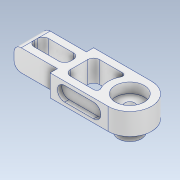
# Autodesk Inventor part: ServoArm
Saved by Autodesk Inventor 2020 (Build 240168000, 168)
## iProperties
Created: 2019-12-15
Part Number: ServoArm
Material: Aluminum 6061
Document SubType Name: Modeling
Designer: Kjell
Density: 2.7 g/cm^3
Appearance: Aluminum - Flat
Author: Kjell
Autodesk Inventor part; units mm, degrees
ref_plane "YZ Plane" through (0, 0, 0) normal (1, 0, 0) x (0, 1, 0)
ref_plane "XZ Plane" through (0, 0, 0) normal (0, 1, 0) x (-1, 0, 0)
ref_plane "XY Plane" through (0, 0, 0) normal (0, 0, 1) x (1, 0, 0)
ref_plane "Work Plane1" through (0, 0, 0) normal (0, 0, 1) x (1, 0, 0)
sketch "Sketch1" plane through (0, 0, 0) normal (0, 0, 1) x (1, 0, 0)
  arc A0 (-2.5, 4.5) -> (-4.5, 2.5) centre (-2.5, 2.5) ccw projected
  arc A1 (-2.5, 4.5) -> (-4.5, 2.5) centre (-2.5, 2.5) ccw projected
  line L0 (-2.5, 4.5) -> (2.5, 4.5) projected
  arc A2 (4.5, 2.5) -> (2.5, 4.5) centre (2.5, 2.5) ccw projected
  line L1 (4.5, 2.5) -> (4.5, -2.5) projected
  arc A3 (2.5, -4.5) -> (4.5, -2.5) centre (2.5, -2.5) ccw projected
  line L2 (2.5, -4.5) -> (-2.5, -4.5) projected
  arc A4 (-4.5, -2.5) -> (-2.5, -4.5) centre (-2.5, -2.5) ccw projected
  line L3 (-4.5, -2.5) -> (-4.5, 2.5) projected
  circle A5 centre (0, 0) radius 5.675 projected
  circle A6 centre (0, 0) radius 8
  circle A7 centre (0, 0) radius 6
  line L4 (-4.55, 2.5) -> (-4.55, -2.5)
  arc A8 (-4.55, -2.5) -> (-2.5, -4.55) centre (-2.5, -2.5) ccw
  line L5 (-2.5, -4.55) -> (2.5, -4.55)
  arc A9 (2.5, -4.55) -> (4.55, -2.5) centre (2.5, -2.5) ccw
  line L6 (4.55, -2.5) -> (4.55, 2.5)
  arc A10 (4.55, 2.5) -> (2.5, 4.55) centre (2.5, 2.5) ccw
  line L7 (2.5, 4.55) -> (-2.5, 4.55)
  point P0 (0, 0)
  dimension "d0" = 16
  dimension "d1" = 12
  dimension "d2" = 0.05
  constraints: 8 end point, 6 point on circle, 5 centre point, 2 coincident, 6 other
  measures "d0" diameter of A6
  measures "d1" diameter of A7
  measures "d2" distance between parallel lines of L2 L5
extrude "Extrusion1" add sketch "Sketch1" against normal blind 5 contours A5 | A6 | A7
sketch "Sketch2" plane through (0, 0, -5) normal (0, 0, -1) x (-1, 0, 0)
  circle A0 centre (0, 0) radius 8 projected
  circle A1 centre (0, 0) radius 6
  dimension "d5" = 12
  constraints: 1 centre point, 1 coincident
  measures "d5" diameter of A1
extrude "Extrusion2" add sketch "Sketch2" along normal blind 3
sketch "Sketch4" plane through (0, 0, 0) normal (0, 0, 1) x (1, 0, 0)
  circle A0 centre (0, 0) radius 8 projected
  arc A1 (0, -15) -> (0, 15) centre (0, 0) ccw
  line L0 (-70, -15) -> (0, -15)
  line L1 (0, 15) -> (-70, 15)
  line L2 (-70, 15) -> (-70, -15)
  line L3 (-30, -67.5) -> (30, -67.5) construction
  line L4 (30, -67.5) -> (30, 67.5) construction
  line L5 (30, 67.5) -> (-30, 67.5) construction
  line L6 (-30, 67.5) -> (-30, -67.5) construction
  line L7 (-30, -67.5) -> (30, 67.5) construction
  line L8 (30, -67.5) -> (-30, 67.5) construction
  dimension "d10" = 30
  dimension "d11" = 60
  dimension "d12" = 135
  dimension "ArmLength" = 70
  constraints: 18 end point, 3 parallel, 2 coincident, 2 horizontal, 2 midpoint, 2 point on circle, 2 tangent, 1 centre point, 1 perpendicular
  measures "d10" diameter of A1
  measures "d11" distance of L5.end L4.end
  measures "d12" distance of L4.end L3.end
  measures "ArmLength" distance from line of L2 A0.centre
extrude "Extrusion4" add sketch "Sketch4" along normal blind 15 contours A0 | L0 L2 L1 A1
sketch "Sketch5" plane through (0, 0, 15) normal (0, 0, 1) x (1, 0, 0)
  arc A0 (0, -15) -> (0, 15) centre (0, 0) ccw projected
  circle A1 centre (0, 0) radius 10
  dimension "d16" = 20
  constraints: 1 centre point, 1 coincident
  measures "d16" diameter of A1
extrude "Extrusion5" cut sketch "Sketch5" against normal blind 7
sketch "Sketch6" plane through (0, 0, 15) normal (0, 0, 1) x (1, 0, 0)
  circle A0 centre (0, 0) radius 10 projected
  arc A1 (0, -15) -> (0, 15) centre (0, 0) ccw projected
  line L0 (-70, 15) -> (-70, -15) projected
  line L1 (-70, -15) -> (0, -15) projected
  line L2 (0, 0) -> (-74.0683, 0) construction
  line L3 (-61, -5) -> (-44, -5)
  line L4 (-40, -1) -> (-40, 1)
  line L5 (-44, 5) -> (-61, 5)
  line L6 (-65, 1) -> (-65, -1)
  line L7 (-65, -5) -> (-40, 5) construction
  line L8 (-40, -5) -> (-65, 5) construction
  line L9 (-31, -10) -> (-14.8625, -10)
  line L10 (-14.8625, 10) -> (-31, 10)
  line L11 (-35, 6) -> (-35, -6)
  line L12 (-35, -10) -> (-11.0172, 10) construction
  line L13 (-11.0172, -10) -> (-35, 10) construction
  arc A2 (-13.1014, 7.0521) -> (-13.1014, -7.0521) centre (0, 0) ccw
  arc A3 (-65, -1) -> (-61, -5) centre (-61, -1) ccw
  arc A4 (-61, 5) -> (-65, 1) centre (-61, 1) ccw
  arc A5 (-40, 1) -> (-44, 5) centre (-44, 1) ccw
  arc A6 (-44, -5) -> (-40, -1) centre (-44, -1) ccw
  arc A7 (-35, -6) -> (-31, -10) centre (-31, -6) ccw
  arc A8 (-31, 10) -> (-35, 6) centre (-31, 6) ccw
  arc A9 (-13.1014, 7.0521) -> (-14.8625, 10) centre (-14.8625, 8) ccw
  arc A10 (-14.8625, -10) -> (-13.1014, -7.0521) centre (-14.8625, -8) ccw
  point P0 (-52.5, 0)
  point P1 (-23.0086, 0)
  dimension "d19" = 25
  dimension "d20" = 10
  dimension "d21" = 20
  dimension "d23" = 5
  dimension "d24" = 5
  dimension "d25" = 4
  dimension "d26" = 2
  constraints: 25 end point, 20 point on circle, 16 point on line, 16 tangent, 9 centre point, 6 equal radius, 4 midpoint, 3 horizontal, 3 parallel, 1 coincident, 1 perpendicular
  measures "d19" distance of L8.end L7.end
  measures "d20" distance of L7.end L8.start
  measures "d21" distance of L12.end L13.start
  measures "d23" distance between parallel lines of L0 L6
  measures "d24" distance between parallel lines of L11 L4
  measures "d25" radius of A3
  measures "d26" radius of A9
extrude "Extrusion6" cut sketch "Sketch6" against normal up to next contours A3 L6 A4 L5 A5 L4 A6 L3 | A7 L11 A8 L10 A9 A2 A10 L9
sketch "Sketch7" plane through (-70, -15, 0) normal (0, -1, 0) x (1, 0, 0)
  line L0 (0, 0) -> (70, 0) projected
  line L1 (0, 15) -> (70, 15) projected
  line L2 (0, 0) -> (0, 15) projected
  line L3 (30, 15) -> (30, 0)
  dimension "d29" = 30
  constraints: 2 end point, 2 point on line, 1 perpendicular
  measures "d29" distance between parallel lines of L3 L2
extrude "Extrusion7" cut sketch "Sketch7" against normal blind 5
mirror "Mirror1" about plane through (0, 0, 0) normal (0, 1, 0) of "Extrusion7"
fillet "Fillet1" radius 5 2 edges at (-70, 0, 15) (-70, 0, 0)
sketch "Sketch8" plane through (0, -15, 0) normal (0, -1, 0) x (1, 0, 0)
  line L0 (0, 0) -> (0, 15) projected
  line L1 (-40, 15) -> (0, 15) projected
  line L2 (-30, 7.5) -> (-10, 7.5) construction
  line L3 (-30, 2.5) -> (-10, 2.5)
  line L4 (-10, 12.5) -> (-30, 12.5)
  arc A0 (-30, 12.5) -> (-30, 2.5) centre (-30, 7.5) ccw
  arc A1 (-10, 2.5) -> (-10, 12.5) centre (-10, 7.5) ccw
  point P0 (-20, 7.5)
  point P1 (0, 7.5)
  point P2 (-20, 15)
  dimension "d33" = 10
  dimension "d34" = 20
  constraints: 8 end point, 4 point on circle, 4 tangent, 3 midpoint, 2 centre point, 1 horizontal alignment, 1 parallel, 1 vertical alignment
  measures "d33" diameter of A1
  measures "d34" distance of L2.end L2.start
extrude "Extrusion8" cut sketch "Sketch8" against normal blind 3
mirror "Mirror2" about plane through (0, 0, 0) normal (0, 1, 0) of "Extrusion8"
sketch "Sketch9" plane through (0, 0, 8) normal (0, 0, 1) x (1, 0, 0)
  circle A0 centre (0, 0) radius 10 projected
  constraints: 1 coincident
ref_plane "Work Plane2" through (0, 0, 0) normal (0, 1, 0) x (-1, 0, 0)
sketch "Sketch10" plane through (0, 0, 8) normal (0, 0, 1) x (1, 0, 0)
  point P0 (0, 0)
  point P1 (0, 0)
hole "Hole1" at (0, 0, 8) at (0, 0, 8) direction (0, 0, -1) diameter 6.6 depth 8
body "Solid1"
